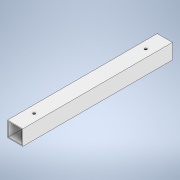
# Autodesk Inventor part: Cablecanal Ranurado 30x30 L=100 mm
Saved by Autodesk Inventor 2020 (Build 240168000, 168)
## iProperties
Created: 2020-07-11
Part Number: Cablecanal Ranurado 30x30 L=100 mm
Material: PPS Plastic
Document SubType Name: Modeling
Designer: Hernan
Density: 1.637 g/cm^3
Appearance: Smooth - White
Author: Hernan
Autodesk Inventor part; units mm, degrees
ref_plane "YZ Plane" through (0, 0, 0) normal (1, 0, 0) x (0, 1, 0)
ref_plane "XZ Plane" through (0, 0, 0) normal (0, 1, 0) x (-1, 0, 0)
ref_plane "XY Plane" through (0, 0, 0) normal (0, 0, 1) x (1, 0, 0)
sketch "Sketch1" plane through (0, 0, 0) normal (0, 0, 1) x (1, 0, 0)
  line L0 (-11.9963, 7.4108) -> (18.0037, 7.4108)
  line L1 (18.0037, 7.4108) -> (18.0037, -22.5892)
  line L2 (18.0037, -22.5892) -> (-11.9963, -22.5892)
  line L3 (-11.9963, -22.5892) -> (-11.9963, 7.4108)
  line L4 (16.3037, 5.7108) -> (-10.2963, 5.7108)
  line L5 (-10.2963, 5.7108) -> (-10.2963, -20.8892)
  line L6 (-10.2963, -20.8892) -> (16.3037, -20.8892)
  line L7 (16.3037, -20.8892) -> (16.3037, 5.7108)
  point P0 (0, 0)
  dimension "d0" = 30
  dimension "d1" = 30
  dimension "d2" = 1.7
  constraints: 16 end point, 4 parallel, 2 perpendicular, 1 horizontal, 3 other
  measures "d0" distance of L0.start L0.end
  measures "d1" distance of L0.end L1.end
  measures "d2" distance between parallel lines of L0 L4
extrude "Extrusion1" add sketch "Sketch1" against normal blind 294.879 contours L0 L1 L2 L3 | L7 L6 L5 L4
extrude "Extrusion2" cut sketch "Sketch1" against normal blind 284.072 contours L7 L6 L5 L4
sketch "Boceto2" plane through (-11.9963, 7.4108, 0) normal (0, 1, 0) x (1, 0, 0)
  line L0 (0, 294.879) -> (30, 294.879) projected
  line L1 (28.3, 0) -> (1.7, 0) projected
  circle A0 centre (15, 37.3509) radius 2.5
  circle A1 centre (15, 257.3509) radius 2.5
  point P0 (11.9963, 0)
  dimension "d7" = 5
  dimension "d8" = 5
  dimension "d12" = 220
  constraints: 2 centre point
  measures "d7" diameter of A0
  measures "d8" diameter of A1
  measures "d12" distance of A0.centre A1.centre
extrude "Extrusión3" cut sketch "Boceto2" against normal blind 10
body "Solid1"
